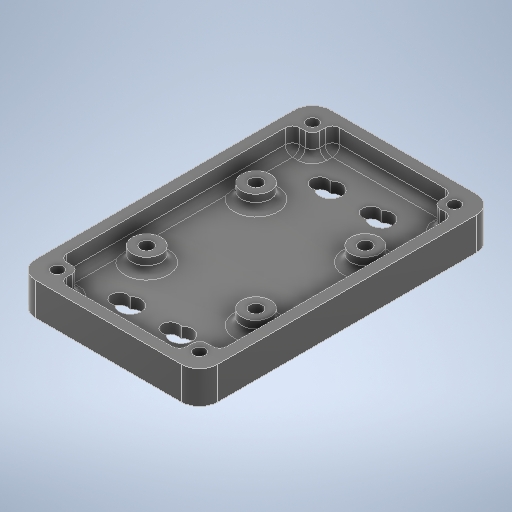
# Autodesk Inventor part: LowerCase
Saved by Autodesk Inventor 2025 (Build 290162010, 162A)
## iProperties
Created: 2025-11-03
Part Number: LowerCase
Material: Genérico
Document SubType Name: Modeling
Designer: João Vitor
Density: 1 g/cm^3
Appearance: Suave - Preto
Author: João Vitor
Autodesk Inventor part; units mm, degrees
ref_plane "YZ Plane" through (0, 0, 0) normal (1, 0, 0) x (0, 1, 0)
ref_plane "XZ Plane" through (0, 0, 0) normal (0, 1, 0) x (-1, 0, 0)
ref_plane "XY Plane" through (0, 0, 0) normal (0, 0, 1) x (1, 0, 0)
sketch "Esboço1" plane through (0, 0, 0) normal (0, 1, 0) x (-1, 0, 0)
  line L0 (-20, 37.5) -> (20, 37.5)
  line L1 (22, 35.5) -> (22, -35.5)
  line L2 (20, -37.5) -> (-20, -37.5)
  line L3 (-22, -35.5) -> (-22, 35.5)
  circle A0 centre (-15, 15) radius 4
  circle A1 centre (-15, -15) radius 4
  circle A2 centre (15, -15) radius 4
  circle A3 centre (15, 15) radius 4
  circle A4 centre (-15, 15) radius 1.75
  circle A5 centre (-15, -15) radius 1.75
  circle A6 centre (15, -15) radius 1.75
  circle A7 centre (15, 15) radius 1.75
  arc A8 (22, 35.5) -> (20, 37.5) centre (20, 35.5) ccw
  arc A9 (20, -37.5) -> (22, -35.5) centre (20, -35.5) ccw
  arc A10 (-22, -35.5) -> (-20, -37.5) centre (-20, -35.5) ccw
  arc A11 (-20, 37.5) -> (-22, 35.5) centre (-20, 35.5) ccw
  line L4 (-20, 40.5) -> (20, 40.5)
  line L5 (25, 35.5) -> (25, -35.5)
  line L6 (20, -40.5) -> (-20, -40.5)
  line L7 (-25, -35.5) -> (-25, 35.5)
  line L8 (-25, 40.5) -> (25, -40.5) construction
  line L9 (25, 40.5) -> (-25, -40.5) construction
  arc A12 (-25, -35.5) -> (-20, -40.5) centre (-20, -35.5) ccw
  arc A13 (-20, 40.5) -> (-25, 35.5) centre (-20, 35.5) ccw
  arc A14 (25, 35.5) -> (20, 40.5) centre (20, 35.5) ccw
  arc A15 (20, -40.5) -> (25, -35.5) centre (20, -35.5) ccw
  circle A16 centre (7, 27.5) radius 3
  circle A17 centre (-7, 27.5) radius 3
  circle A18 centre (10, 27.5) radius 2.25
  circle A19 centre (-4, 27.5) radius 2.25
  circle A20 centre (10, -27.5) radius 2.25
  circle A21 centre (-4, -27.5) radius 2.25
  circle A22 centre (7, -27.5) radius 3
  circle A23 centre (-7, -27.5) radius 3
  circle A24 centre (19.5, 35) radius 1.6
  circle A25 centre (-19.5, 35) radius 1.6
  circle A26 centre (-19.5, -35) radius 1.6
  circle A27 centre (19.5, -35) radius 1.6
  line L10 (-16.5, 37.5) -> (-16.5, 34)
  line L11 (-18.5, 32) -> (-22, 32)
  line L12 (16.5, 37.5) -> (16.5, 34)
  line L13 (18.5, 32) -> (22, 32)
  line L14 (22, -32) -> (18.5, -32)
  line L15 (16.5, -34) -> (16.5, -37.5)
  line L16 (-22, -32) -> (-18.5, -32)
  line L17 (-16.5, -34) -> (-16.5, -37.5)
  arc A28 (16.5, 34) -> (18.5, 32) centre (18.5, 34) ccw
  arc A29 (-18.5, 32) -> (-16.5, 34) centre (-18.5, 34) ccw
  arc A30 (18.5, -32) -> (16.5, -34) centre (18.5, -34) ccw
  arc A31 (-16.5, -34) -> (-18.5, -32) centre (-18.5, -34) ccw
  point P0 (-11, 15)
  point P1 (-12, 37.5)
  point P2 (-15, 11)
  point P3 (-22, 12.8923)
  point P4 (-15, -11)
  point P5 (-22, -11.1077)
  point P6 (-11, -15)
  point P7 (-12, -37.5)
  point P8 (11.3796, -16.7007)
  point P9 (12, -37.5)
  point P10 (15, -11)
  point P11 (22, -11.1077)
  point P12 (15, 11)
  point P13 (22, 12.8923)
  point P14 (11, 15)
  point P15 (12, 37.5)
  point P16 (-4.8438, -25.4142)
  point P17 (-4.8438, -29.5858)
  point P18 (9.1563, -25.4142)
  point P19 (9.1562, -29.5858)
  point P20 (-4.8438, 29.5858)
  point P21 (-4.8438, 25.4142)
  point P22 (9.1563, 29.5858)
  point P23 (9.1562, 25.4142)
  point P24 (0, 0)
  point P25 (0, 0)
  point P26 (-16.5, 32)
  point P27 (-20.25, 32)
  point P28 (16.5, 32)
  point P29 (16.5, -32)
  point P30 (-16.5, -32)
  dimension "d37" = 6
  dimension "d38" = 6
  dimension "d45" = 6
  dimension "d46" = 6
  dimension "d2" = 8
  dimension "d7" = 3.5
  dimension "d8" = 2
  dimension "d9" = 3
  dimension "d10" = 3
  dimension "d11" = 5
  dimension "d28" = 30
  dimension "d30" = 44
  dimension "d31" = 75
  dimension "d33" = 30
  dimension "d35" = 3
  dimension "d36" = 3
  dimension "d39" = 4.5
  dimension "d40" = 4.5
  dimension "d44" = 10
  dimension "d47" = 4.5
  dimension "d48" = 4.5
  dimension "d53" = 10
  dimension "d54" = 15
  dimension "d55" = 15
  dimension "d56" = 7
  dimension "d57" = 7
  dimension "d58" = 7
  dimension "d59" = 7
  dimension "d62" = 2.5
  dimension "d63" = 2.5
  dimension "d64" = 2.5
  dimension "d65" = 2.5
  dimension "d66" = 3
  dimension "d67" = 3
  dimension "d70" = 3.2
  dimension "d71" = 3
  dimension "d72" = 3
  dimension "d73" = 2
  dimension "d74" = 2
  dimension "d76" = 10
  dimension "d77" = 4
  constraints: 36 end point, 32 point on circle, 32 point on line, 28 centre point, 24 tangent, 17 equal radius, 12 horizontal alignment, 6 perpendicular, 6 vertical alignment, 4 concentric, 4 horizontal, 4 parallel, 3 midpoint, 2 vertical, 13 other
  measures "d2" diameter of A3
  measures "d7" diameter of A4
  measures "d8" radius of A8
  measures "d9" distance between parallel lines of L0 L4
  measures "d10" distance between parallel lines of L5 L1
  measures "d11" radius of A12
  measures "d28" distance of A1.centre A0.centre
  measures "d30" distance between parallel lines of L1 L3
  measures "d31" distance between parallel lines of L2 L0
  measures "d33" distance of A7.centre A4.centre
  measures "d35" distance between parallel lines of L3 L7
  measures "d36" distance between parallel lines of L2 L6
  measures "d39" diameter of A18
  measures "d40" diameter of A19
  measures "d44" distance from line of L0 point (-7, 27.5)
  measures "d47" diameter of A20
  measures "d48" diameter of A21
  measures "d53" distance from line of L2 point (-7, -27.5)
  measures "d54" horizontal distance of point (0, 0) A0.centre
  measures "d55" horizontal distance of point (0, 0) A1.centre
  measures "d56" horizontal distance of point (0, 0) point (-7, -27.5)
  measures "d57" horizontal distance of point (0, 0) point (7, -27.5)
  measures "d58" horizontal distance of point (0, 0) point (-7, 27.5)
  measures "d59" horizontal distance of point (0, 0) point (7, 27.5)
  measures "d62" distance from line of L0 A24.centre
  measures "d63" distance from line of L3 A26.centre
  measures "d64" distance from line of L1 A24.centre
  measures "d65" distance from line of L2 A26.centre
  measures "d66" vertical distance of A25.centre point (-20.25, 32)
  measures "d67" distance from line of L10 A25.centre
  measures "d70" diameter of A24
  measures "d71" distance from line of A27.centre L15
  measures "d72" distance from line of A27.centre L14
  measures "d73" radius of A28
  measures "d74" radius of A30
  measures "d76" horizontal distance of point (0, 0) A20.centre
  measures "d77" horizontal distance of point (0, 0) A21.centre
extrude "Extrusão1" add sketch "Esboço1" along normal blind 3 contours L0 L10 A29 L11 L3 A11 | L0 L12 A28 L13 L1 L14 A30 L15 L2 L17 A31 L16 L3 L11 A29 L10 | L0 A8 L1 L13 A28 L12 | L16 A31 L17 L2 A10 L3 | L1 A9 L2 L15 A30 L14 | A0 | A1 | A2 | A3 | A4 | A5 | A6 | A7 | A16 A18 | A16 A18 | A18 A16 | A17 A19 | A17 A19 | A19 A17 | A20 A22 | A22 A20 | A20 A22 | A21 A23 | A23 A21 | A21 A23 | A24 | A25 | A26 | A27
extrude "Extrusão2" add sketch "Esboço1" along normal blind 7 contours A0 | A1 | A2 | A3
extrude "Extrusão3" add sketch "Esboço1" along normal blind 9 contours L4 A14 L5 A15 L6 A12 L7 A13
extrude "Extrusão4" cut sketch "Esboço1" along normal blind 3.5 contours A16 A18 | A16 A18 | A18 A16 | A17 A19 | A17 A19 | A19 A17 | A20 A22 | A22 A20 | A20 A22 | A21 A23 | A23 A21 | A21 A23
fillet "Arredondamento1" radius 2 12 edges at (-21.4142, 3, 36.9142) (0, 3, 37.5) (21.4142, 3, 36.9142) (22, 3, 0) (21.4142, 3, -36.9142) (0, 3, -37.5) (-21.4142, 3, -36.9142) (-22, 3, 0) (-11, 3, 15) (19, 3, 15) (19, 3, -15) (-11, 3, -15)
extrude "Extrusão6" add sketch "Esboço1" along normal blind 9 contours L0 L10 A29 L11 L3 A11 | L0 A8 L1 L13 A28 L12 | L16 A31 L17 L2 A10 L3 | L1 A9 L2 L15 A30 L14
fillet "Arredondamento2" radius 2 28 edges at (-16.5, 7, 37.5) (-16.5, 3, 34.75) (-17.0858, 3, 32.5858) (-19.25, 3, 32) (-21.4142, 3.5858, 32) (-22, 7, 32) (-16.5, 3.5858, 36.9142) (19.25, 3, 32) (21.4142, 3.5858, 32) (22, 7, 32) (16.5, 3, 34.75) (16.5, 3.5858, 36.9142) (16.5, 7, 37.5) (17.0858, 3, 32.5858) (-19.25, 3, -32) (-21.4142, 3.5858, -32) (-22, 7, -32) (-16.5, 3, -34.75) (-16.5, 3.5858, -36.9142) (-16.5, 7, -37.5) (-17.0858, 3, -32.5858) (16.5, 3.5858, -36.9142) (16.5, 7, -37.5) (17.0858, 3, -32.5858) (19.25, 3, -32) (21.4142, 3.5858, -32) (22, 7, -32) (16.5, 3, -34.75)
equation "\"d24\" = d18"
equation "\"d18\" = 3.5"
